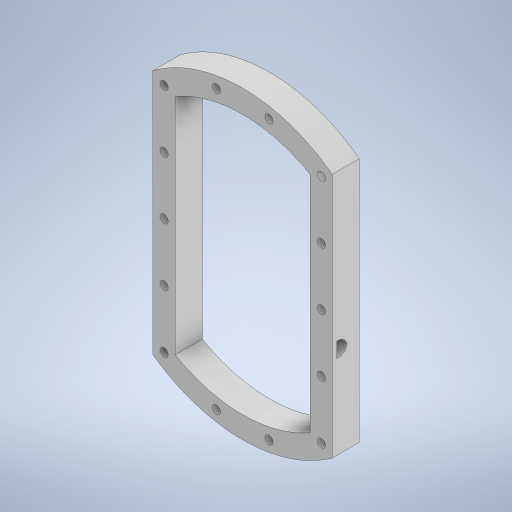
# Autodesk Inventor part: new_retainer_full_cap
Saved by Autodesk Inventor 2023 (Build 270158000, 158)
## iProperties
Created: 2022-07-28
Part Number: new_retainer_full_cap
Material: Generic
Document SubType Name: Modeling
Designer: djp6984
Density: 1 g/cm^3
Appearance: Default
Author: djp6984
Autodesk Inventor part; units mm, degrees
ref_plane "YZ Plane" through (0, 0, 0) normal (1, 0, 0) x (0, 1, 0)
ref_plane "XZ Plane" through (0, 0, 0) normal (0, 1, 0) x (-1, 0, 0)
ref_plane "XY Plane" through (0, 0, 0) normal (0, 0, 1) x (1, 0, 0)
sketch "Sketch1" plane through (0, 0, 0) normal (0, 0, 1) x (1, 0, 0)
  arc A0 (25.273, 34.559) -> (0.0081, 42.8141) centre (0, 0) ccw
  line L0 (25.273, 34.559) -> (25.273, 0)
  line L1 (18.923, 0) -> (18.923, 31.5055)
  arc A1 (18.923, 31.5055) -> (0.0081, 36.4641) centre (-0.083, -2.439) ccw
  arc A2 (23.2283, 0) -> (20.9677, 0) centre (22.098, 0) ccw
  circle A3 centre (22.098, 32.4528) radius 1.1303
  circle A4 centre (22.098, 16.1968) radius 1.1303
  circle A5 centre (7.372, 39.0479) radius 1.1303
  arc A6 (-20.9677, 0) -> (-23.2283, 0) centre (-22.098, 0) ccw
  circle A7 centre (-22.098, 16.1968) radius 1.1303
  circle A8 centre (-22.098, 32.4528) radius 1.1303
  circle A9 centre (-7.372, 39.0479) radius 1.1303
  arc A10 (-0.0081, 36.4641) -> (-18.923, 31.5055) centre (0.083, -2.439) ccw
  arc A11 (-0.0081, 42.8141) -> (-25.273, 34.559) centre (0, 0) ccw
  line L2 (-25.273, 34.559) -> (-25.273, 0)
  line L3 (-18.923, 0) -> (-18.923, 31.5055)
  line L4 (25.273, -34.559) -> (25.273, 0)
  arc A12 (0.0081, -42.8141) -> (25.273, -34.559) centre (0, 0) ccw
  arc A13 (-25.273, -34.559) -> (-0.0081, -42.8141) centre (0, 0) ccw
  line L5 (-25.273, -34.559) -> (-25.273, 0)
  line L6 (-18.923, 0) -> (-18.923, -31.5055)
  arc A14 (-18.923, -31.5055) -> (-0.0081, -36.4641) centre (0.083, 2.439) ccw
  arc A15 (0.0081, -36.4641) -> (18.923, -31.5055) centre (-0.083, 2.439) ccw
  line L7 (18.923, 0) -> (18.923, -31.5055)
  arc A16 (-23.2283, 0) -> (-20.9677, 0) centre (-22.098, 0) ccw
  circle A17 centre (-22.098, -16.1968) radius 1.1303
  circle A18 centre (-22.098, -32.4528) radius 1.1303
  circle A19 centre (-7.372, -39.0479) radius 1.1303
  circle A20 centre (7.372, -39.0479) radius 1.1303
  circle A21 centre (22.098, -32.4528) radius 1.1303
  circle A22 centre (22.098, -16.1968) radius 1.1303
  arc A23 (20.9677, 0) -> (23.2283, 0) centre (22.098, 0) ccw
  point P0 (0, 29.76)
  point P1 (9.9838, 29.1027)
  point P2 (9.9839, 22.365)
  point P3 (9.9841, 15.6273)
  point P4 (9.9842, 8.8896)
  point P5 (9.9844, 2.1519)
  point P6 (-17.2373, 0)
  point P7 (-17.2389, 0)
  point P8 (-17.2362, -2.4348)
  point P9 (9.9845, -4.5858)
  point P10 (9.9847, -11.3235)
  point P11 (9.9848, -18.0612)
  point P12 (9.9849, -24.7989)
  point P13 (-0.4822, -30.8495)
  point P14 (0, -28.8424)
  point P15 (-10.2647, -28.1682)
  point P16 (-10.2649, -21.4305)
  point P17 (-10.265, -14.6929)
  point P18 (-10.2652, -7.9552)
  point P19 (-10.2653, -1.2175)
  point P20 (-10.2655, 5.5201)
  point P21 (-10.2656, 12.2578)
  point P22 (-10.2657, 18.9955)
  point P23 (-10.2659, 25.7332)
  point P24 (0.294, 31.7784)
  dimension "d1" = 6.35
  dimension "d2" = 2.2606
  dimension "d3" = 2.2606
  dimension "d4" = 2.2606
  dimension "d6" = 2.2606
  constraints: 24 centre point, 24 point on circle, 16 end point, 2 vertical
  measures "d1" distance between parallel lines of L1 L0
  measures "d2" diameter of A2
  measures "d3" diameter of A3
  measures "d4" diameter of A4
  measures "d6" diameter of A5
sketch "Sketch4" plane through (0, 0, 0) normal (0, 0, 1) x (1, 0, 0)
  line L0 (-18.985, 31.3156) -> (-18.985, -31.5153)
  line L1 (18.8873, 31.3156) -> (18.8873, -31.5153)
  line L2 (-25.3178, 34.4199) -> (-25.3178, -34.6195)
  line L3 (25.0959, 34.4199) -> (25.0959, -34.6195)
  arc A0 (18.8873, 31.3156) -> (-18.985, 31.3156) centre (-0.0488, -1.3553) ccw
  arc A1 (-18.985, -31.5153) -> (18.8873, -31.5153) centre (-0.0488, 1.0453) ccw
  arc A2 (25.0959, 34.4199) -> (-25.3178, 34.4199) centre (-0.1109, 0.7967) ccw
  arc A3 (-25.3178, -34.6195) -> (25.0959, -34.6195) centre (-0.1109, 0.3555) ccw
  point P0 (0, 0)
  constraints: 8 end point, 8 point on circle, 4 centre point, 3 vertical, 1 parallel
extrude "Extrusion1" add sketch "Sketch4" along normal blind 7.62
extrude "Extrusion2" cut sketch "Sketch1" along normal blind 7.62
sketch "Sketch5" plane through (25.0959, -34.6195, 0) normal (1, 0, 0) x (0, 0, -1)
  line L0 (-7.62, 3.1043) -> (-7.62, 65.9351) projected
  line L1 (-6.35, 27.8057) -> (-6.0293, 27.8057)
  line L2 (-3.4893, 25.2657) -> (-3.4893, 26.1098)
  line L3 (-6.0293, 23.5698) -> (-6.35, 23.5698)
  line L4 (-6.35, 23.5698) -> (-6.35, 27.8057)
  arc A0 (-3.4893, 25.2657) -> (-6.0293, 27.8057) centre (-6.0293, 25.2657) ccw
  arc A1 (-6.0293, 23.5698) -> (-3.4893, 26.1098) centre (-6.0293, 26.1098) ccw
  point P0 (0, 34.6195)
  point P1 (-3.5246, 25.6877)
  dimension "d16" = 2.54
  dimension "d17" = 1.27
  constraints: 8 end point, 4 point on circle, 4 tangent, 2 centre point, 2 parallel, 1 equal radius, 1 horizontal, 1 perpendicular
  measures "d16" radius of A0
  measures "d17" distance between parallel lines of L0 L4
extrude "Extrusion3" cut sketch "Sketch5" against normal blind 12.7 contours L1 A0 A1 L3 L4
body "Solid1"
